Autodesk Fusion 360 part; units mm, degrees
note: some values were not read from the file. Chosen so that the rebuilt part matches the saved one: which bodies a step acts on.
(part 2 of 2)
sketch "Sketch2 (3)" plane through (0, 2, 0) normal (0, 1, 0) x (-1, 0, 0) in component "RFIDShelf"
  circle A0 centre (-31.35, -184.4) radius 3.25
  line L0 (-4, -4.6) -> (-58.7, -4.6)
  line L1 (-58.7, -4.6) -> (-62.7, -8.6)
  line L2 (-62.7, -8.6) -> (-62.7, -50.6)
  line L3 (-62.7, -50.6) -> (-58.7, -54.6)
  line L4 (-58.7, -54.6) -> (-60.7, -54.6)
  line L5 (-60.7, -54.6) -> (-60.7, -95.2)
  line L6 (-60.7, -95.2) -> (-58.7, -95.2)
  line L7 (-58.7, -95.2) -> (-62.7, -99.2)
  line L8 (-62.7, -99.2) -> (-62.7, -111.2)
  line L9 (-62.7, -111.2) -> (-58.7, -115.2)
  line L10 (-58.7, -115.2) -> (-60.7, -115.2)
  line L11 (-60.7, -115.2) -> (-60.7, -119.8)
  line L12 (-60.7, -119.8) -> (-58.7, -119.8)
  line L13 (-58.7, -119.8) -> (-62.7, -123.8)
  line L14 (-62.7, -123.8) -> (-62.7, -145.8)
  line L15 (-62.7, -145.8) -> (-58.7, -149.8)
  line L16 (-58.7, -149.8) -> (-60.7, -149.8)
  line L17 (-60.7, -149.8) -> (-60.7, -154.4)
  line L18 (-60.7, -154.4) -> (-58.7, -154.4)
  line L19 (-58.7, -154.4) -> (-62.7, -158.4)
  line L20 (-62.7, -158.4) -> (-62.7, -214.4)
  line L21 (-62.7, -214.4) -> (0, -214.4)
  line L22 (0, -214.4) -> (0, -158.4)
  line L23 (0, -158.4) -> (-4, -154.4)
  line L24 (-4, -154.4) -> (-2, -154.4)
  line L25 (-2, -154.4) -> (-2, -149.8)
  line L26 (-2, -149.8) -> (-4, -149.8)
  line L27 (-4, -149.8) -> (0, -145.8)
  line L28 (0, -145.8) -> (0, -123.8)
  line L29 (0, -123.8) -> (-4, -119.8)
  line L30 (-4, -119.8) -> (-2, -119.8)
  line L31 (-2, -119.8) -> (-2, -115.2)
  line L32 (-2, -115.2) -> (-4, -115.2)
  line L33 (-4, -115.2) -> (0, -111.2)
  line L34 (0, -111.2) -> (0, -99.2)
  line L35 (0, -99.2) -> (-4, -95.2)
  line L36 (-4, -95.2) -> (-2, -95.2)
  line L37 (-2, -95.2) -> (-2, -54.6)
  line L38 (-2, -54.6) -> (-4, -54.6)
  line L39 (-4, -54.6) -> (0, -50.6)
  line L40 (0, -50.6) -> (0, -8.6)
  line L41 (0, -8.6) -> (-4, -4.6)
  line L42 (-4, -149.8) -> (-58.7, -149.8) construction
  line L43 (-2.2, -149.8) -> (-60.5, -149.8)
  line L44 (-60.5, -149.8) -> (-60.5, -154)
  line L45 (-60.5, -154) -> (-2.2, -154)
  line L46 (-2.2, -154) -> (-2.2, -149.8)
  line L47 (-31.35, -149.8) -> (-31.35, -154) construction
  line L48 (-2.2, -151.9) -> (-4.2, -151.9) construction
  line L49 (-4.2, -149.8) -> (-4.2, -154)
  line L50 (-31.35, -149.8) -> (-31.35, -154) construction
  line L51 (-60.5, -151.9) -> (-58.5, -151.9) construction
  line L52 (-58.5, -154) -> (-58.5, -149.8)
  line L53 (-4.2, -154) -> (-58.5, -154)
  line L54 (-31.35, -154) -> (-52.59, -154) construction
  line L55 (-31.35, -154) -> (-10.11, -154) construction
  line L56 (-52.59, -154) -> (-52.59, -149.8)
  line L57 (-10.11, -154) -> (-10.11, -149.8)
  dimension "d344" = 58.3
  dimension "d345" = 4.2
  dimension "d346" = 2
  dimension "d347" = 4.2
  dimension "d348" = 2
  dimension "d356" = 21.24
  dimension "d357" = 21.24
  constraint coincident L26.end L27.start
  constraint coincident L15.end L16.start
  constraint horizontal L43
  constraint vertical L44
  constraint horizontal L45
  constraint vertical L46
  constraint coincident L42 L43.start
  constraint midpoint L42 L47.start
  constraint midpoint L45 L47.end
  constraint perpendicular L42 L47
  constraint midpoint L46 L48.start
  constraint perpendicular L46 L48
  constraint coincident L43 L49.start
  constraint coincident L45 L49.end
  constraint perpendicular L43 L49
  constraint coincident L48.end L49
  constraint perpendicular L42 L50
  constraint midpoint L44 L51.start
  constraint perpendicular L44 L51
  constraint coincident L45 L52.start
  constraint coincident L42 L52.end
  constraint perpendicular L42 L52
  constraint coincident L51.end L52
  constraint coincident L49 L53.start
  constraint coincident L52 L53.end
  constraint perpendicular L52 L53
  constraint coincident L47.end L53
  constraint coincident L53 L54.end
  constraint coincident L53 L55.end
  constraint coincident L43 L56.end
  constraint coincident L43 L57.end
  constraint perpendicular L42 L57
  constraint perpendicular L43 L56
  measures "d344" distance of L43.start L43.end
  measures "d345" distance of L43.start L45.end
  measures "d346" distance of L48.start L48.end
  measures "d347" distance of L47.start L47.end
  measures "d348" distance of L51.start L51.end
  measures "d356" distance of L47.end L54.end
  measures "d357" distance of L47.end L55.end
extrude "Extrude2''" add sketch "Sketch2 (3)" along normal blind 82.4 separate body contours L26 L43 L45 L46 L49 | L16 L43 L44 L45 L52 | L43 L45 L53 L56 L57 makes body 14 at (58.5, 56.9333, -152.6) makes body 15 at (2.2, 56.9333, -152.6) makes body 16 at (38.43, 29.4667, -154) in component "RFIDShelf"
extrude "Extrude6" add sketch "Sketch2 (3)" along normal blind 10 contours L43 L45 L49 L53 L57 | L43 L45 L52 L53 L56 bodies 14 15 16 in component "RFIDShelf"
extrude "Extrude7'''" add sketch "Sketch2 (3)" against normal blind 10 from surface at 82.4 contours L43 L45 L49 L53 L57 | L43 L45 L52 L53 L56 bodies 14 in component "RFIDShelf"
sketch "Sketch3 (2)" plane through (0, 84.4, 0) normal (0, 1, 0) x (-1, 0, 0) in component "RFIDShelf"
  line L0 (-2.2, -154) -> (-2.2, -149.8)
  line L1 (-2.2, -149.8) -> (-60.5, -149.8)
  line L2 (-60.5, -149.8) -> (-60.5, -154)
  line L3 (-60.5, -154) -> (-2.2, -154)
  line L4 (1.1849, -152.6692) -> (-2.2, -154)
  line L5 (-8.5, -161.5333) -> (-0.9667, -154)
  line L6 (-8.5, -161.5333) -> (-5.8622, -161.5333) construction
  line L7 (-4.2, -154) -> (-58.5, -154)
  dimension "d358" = 45
  constraint coincident L0.start L3.end
  constraint horizontal L6
  constraint coincident L5.end L7
  measures "d358" angle of L5 L6
sketch "Sketch5 (2)" plane through (0, 0, -149.8) normal (0, 0, 1) x (1, 0, 0) in component "RFIDShelf"
  line L0 (2.2, 2) -> (60.5, 2)
  line L1 (52.59, 12) -> (52.59, 74.4)
  line L2 (60.5, 84.4) -> (2.2, 84.4)
  line L3 (10.11, 74.4) -> (10.11, 12)
  line L4 (46.97, 84.4) -> (46.97, 70.87) construction
  line L5 (46.97, 70.87) -> (58.5, 70.87) construction
  line L6 (58.5, 12) -> (58.5, 74.4) construction
  line L7 (26.75, 84.4) -> (26.75, 28.96) construction
  line L8 (26.75, 28.96) -> (58.5, 28.96) construction
  circle A0 centre (26.75, 28.96) radius 1.7
  circle A1 centre (26.75, 28.96) radius 3
  circle A2 centre (46.97, 70.87) radius 3
  circle A3 centre (46.97, 70.87) radius 1.7
  line L9 (10.11, 12) -> (4.2, 12)
  line L10 (4.2, 12) -> (4.2, 74.4)
  line L11 (4.2, 74.4) -> (10.11, 74.4)
  line L12 (2.2, 84.4) -> (2.2, 2)
  line L13 (60.5, 2) -> (60.5, 84.4)
  line L14 (52.59, 74.4) -> (58.5, 74.4)
  line L15 (58.5, 74.4) -> (58.5, 12)
  line L16 (58.5, 12) -> (52.59, 12)
  dimension "d400" = 13.53
  dimension "d401" = 11.53
  dimension "d402" = 55.44
  dimension "d403" = 31.75
  dimension "d404" = 3.4
  dimension "d405" = 6
  dimension "d406" = 6
  dimension "d407" = 3.4
  constraint coincident L2 L4.start
  constraint perpendicular L2 L4
  constraint perpendicular L4 L5
  constraint coincident L5.end L6
  constraint coincident L2 L7.start
  constraint perpendicular L2 L7
  constraint perpendicular L6 L8
  constraint coincident L6 L8.end
  constraint coincident L7.end L8.start
  constraint coincident L4.end L5.start
  constraint concentric A2 A3
  measures "d400" distance of L4.start L4.end
  measures "d401" distance of L4.end L5.end
  measures "d402" distance of L7.start L7.end
  measures "d403" distance of L7.end L8.end
  measures "d404" diameter of A0
  measures "d405" diameter of A1
  measures "d406" diameter of A2
  measures "d407" diameter of A3
extrude "Extrude4" cut sketch "Sketch5 (2)" against normal up to surface (4.2 mm away) contours A0 | A3 bodies 14 in component "RFIDShelf"
extrude "Extrude5" cut sketch "Sketch5 (2)" against normal blind 3.2 contours A1 | A2 bodies 14 in component "RFIDShelf"
sketch "Sketch7" plane through (0, 2, 0) normal (0, 1, 0) x (-1, 0, 0) in component "Main Case"
  circle A0 centre (-31.35, -184.4) radius 3.25
  line L0 (-4, -4.6) -> (-58.7, -4.6)
  line L1 (-58.7, -4.6) -> (-62.7, -8.6)
  line L2 (-62.7, -8.6) -> (-62.7, -50.6)
  line L3 (-62.7, -50.6) -> (-58.7, -54.6)
  line L4 (-58.7, -54.6) -> (-60.7, -54.6)
  line L5 (-60.7, -54.6) -> (-60.7, -95.2)
  line L6 (-60.7, -95.2) -> (-58.7, -95.2)
  line L7 (-58.7, -95.2) -> (-62.7, -99.2)
  line L8 (-62.7, -99.2) -> (-62.7, -111.2)
  line L9 (-62.7, -111.2) -> (-58.7, -115.2)
  line L10 (-58.7, -115.2) -> (-60.7, -115.2)
  line L11 (-60.7, -115.2) -> (-60.7, -119.8)
  line L12 (-60.7, -119.8) -> (-58.7, -119.8)
  line L13 (-58.7, -119.8) -> (-62.7, -123.8)
  line L14 (-62.7, -123.8) -> (-62.7, -145.8)
  line L15 (-62.7, -145.8) -> (-58.7, -149.8)
  line L16 (-58.7, -149.8) -> (-60.7, -149.8)
  line L17 (-60.7, -149.8) -> (-60.7, -154.4)
  line L18 (-60.7, -154.4) -> (-58.7, -154.4)
  line L19 (-58.7, -154.4) -> (-62.7, -158.4)
  line L20 (-62.7, -158.4) -> (-62.7, -214.4)
  line L21 (-62.7, -214.4) -> (0, -214.4)
  line L22 (0, -214.4) -> (0, -158.4)
  line L23 (0, -158.4) -> (-4, -154.4)
  line L24 (-4, -154.4) -> (-2, -154.4)
  line L25 (-2, -154.4) -> (-2, -149.8)
  line L26 (-2, -149.8) -> (-4, -149.8)
  line L27 (-4, -149.8) -> (0, -145.8)
  line L28 (0, -145.8) -> (0, -123.8)
  line L29 (0, -123.8) -> (-4, -119.8)
  line L30 (-4, -119.8) -> (-2, -119.8)
  line L31 (-2, -119.8) -> (-2, -115.2)
  line L32 (-2, -115.2) -> (-4, -115.2)
  line L33 (-4, -115.2) -> (0, -111.2)
  line L34 (0, -111.2) -> (0, -99.2)
  line L35 (0, -99.2) -> (-4, -95.2)
  line L36 (-4, -95.2) -> (-2, -95.2)
  line L37 (-2, -95.2) -> (-2, -54.6)
  line L38 (-2, -54.6) -> (-4, -54.6)
  line L39 (-4, -54.6) -> (0, -50.6)
  line L40 (0, -50.6) -> (0, -8.6)
  line L41 (0, -8.6) -> (-4, -4.6)
  line L42 (-2, -115.2) -> (0, -115.2) construction
  line L43 (0, -115.2) -> (0, -102.2) construction
  line L44 (0, -102.2) -> (-21.5, -102.2)
  line L45 (-21.5, -102.2) -> (-21.5, -121.2)
  line L46 (-21.5, -121.2) -> (0, -121.2)
  line L47 (-20, -61) -> (-43, -61)
  line L48 (-43, -61) -> (-43, -28)
  line L49 (-43, -28) -> (-20, -28)
  line L50 (-20, -28) -> (-20, -61)
  dimension "d504" = 13
  dimension "d505" = 21.5
  dimension "d506" = 19
  constraint coincident L31.end L32.start
  constraint perpendicular L31 L42
  constraint perpendicular L42 L43
  constraint perpendicular L43 L44
  constraint perpendicular L44 L45
  constraint perpendicular L45 L46
  constraint horizontal L47
  constraint vertical L48
  constraint horizontal L49
  constraint vertical L50
  measures "d504" distance of L42.end L43.end
  measures "d505" distance of L43.end L44.end
  measures "d506" distance of L44.end L45.end
extrude "Extrude13" cut sketch "Sketch4" along normal up to surface (2 mm away) contours L4 L13 L19 L34 L35 L36 L38 L58 L59 L62 L65 L66 bodies 1 in component "Main Case"
extrude "Extrude14" cut sketch "Sketch4" along normal blind 2 contours A7 bodies 1 in component "Main Case"
sketch "Sketch8" plane through (0, 2, 0) normal (0, 1, 0) x (-1, 0, 0) in component "Main Case"
  circle A0 centre (-31.35, -74.9) radius 12.5
  line L0 (-4, -54.6) -> (-58.7, -54.6)
  line L1 (-58.7, -54.6) -> (-60.7, -54.6)
  line L2 (-60.7, -54.6) -> (-60.7, -95.2)
  line L3 (-60.7, -95.2) -> (-58.7, -95.2)
  line L4 (-58.7, -95.2) -> (-62.7, -99.2)
  line L5 (-62.7, -99.2) -> (-62.7, -111.2)
  line L6 (-62.7, -111.2) -> (-58.7, -115.2)
  line L7 (-58.7, -115.2) -> (-60.7, -115.2)
  line L8 (-60.7, -115.2) -> (-60.7, -119.8)
  line L9 (-60.7, -119.8) -> (-58.7, -119.8)
  line L10 (-58.7, -119.8) -> (-62.7, -123.8)
  line L11 (-62.7, -123.8) -> (-62.7, -145.8)
  line L12 (-62.7, -145.8) -> (-58.7, -149.8)
  line L13 (-58.7, -149.8) -> (-60.7, -149.8)
  line L14 (-60.7, -149.8) -> (-60.7, -154.4)
  line L15 (-60.7, -154.4) -> (-58.7, -154.4)
  line L16 (-58.7, -154.4) -> (-62.7, -158.4)
  line L17 (-62.7, -158.4) -> (-62.7, -214.4)
  line L18 (-62.7, -214.4) -> (0, -214.4)
  line L19 (0, -214.4) -> (0, -158.4)
  line L20 (0, -158.4) -> (-4, -154.4)
  line L21 (-4, -154.4) -> (-2, -154.4)
  line L22 (-2, -154.4) -> (-2, -149.8)
  line L23 (-2, -149.8) -> (-4, -149.8)
  line L24 (-4, -149.8) -> (0, -145.8)
  line L25 (0, -145.8) -> (0, -123.8)
  line L26 (0, -123.8) -> (-4, -119.8)
  line L27 (-4, -119.8) -> (-2, -119.8)
  line L28 (-2, -119.8) -> (-2, -115.2)
  line L29 (-2, -115.2) -> (-4, -115.2)
  line L30 (-4, -115.2) -> (0, -111.2)
  line L31 (0, -111.2) -> (0, -99.2)
  line L32 (0, -99.2) -> (-4, -95.2)
  line L33 (-4, -95.2) -> (-2, -95.2)
  line L34 (-2, -95.2) -> (-2, -54.6)
  line L35 (-2, -54.6) -> (-4, -54.6)
  circle A1 centre (-31.35, -184.4) radius 3.25
  line L36 (-4, -119.8) -> (-18.2, -119.8)
  line L37 (-18.2, -119.8) -> (-18.2, -104.8)
  line L38 (-18.2, -104.8) -> (-4, -104.8)
  line L39 (-4, -104.8) -> (-4, -119.8)
  dimension "d516" = 14.2
  dimension "d517" = 15
  constraint coincident L26.end L27.start
  constraint parallel L27 L36
  constraint perpendicular L27 L37
  constraint perpendicular L37 L38
  constraint perpendicular L36 L39
  measures "d516" distance of L26.end L36.end
  measures "d517" distance of L36.end L37.end
extrude "Extrude15" cut sketch "Sketch8" against normal blind 2 contours L36 L37 L38 L39 bodies 1 in component "Main Case"
component "Case Attempt 2" placed x (1, 0, 0) y (0, 1, 0) z (0, 0, 1) at (0, 0, 0)
component "Main Case" placed x (1, 0, 0) y (0, 1, 0) z (0, 0, 1) at (0, 0, 0) in component "Case Attempt 2"
component "Case Lid" placed x (1, 0, 0) y (0, 1, 0) z (0, 0, 1) at (0, 0, 0) in component "Case Attempt 2"
component "UnoShelfV2" placed x (1, 0, 0) y (0, 1, 0) z (0, 0, 1) at (0, 0, 0) in component "Case Attempt 2"
component "BatteryShelf" placed x (1, 0, 0) y (0, 1, 0) z (0, 0, 1) at (0, 0, 0) in component "Case Attempt 2"
component "ConverterShelf" placed x (1, 0, 0) y (0, 1, 0) z (0, 0, 1) at (0, 0, 0) in component "Case Attempt 2"
component "RFIDShelf" placed x (1, 0, 0) y (0, 1, 0) z (0, 0, 1) at (0, 0, 0) in component "Case Attempt 2"
equation "thickness = 2 mm"
equation "width = 54.1 mm"
equation "nanoLength = 78.2 mm"
equation "unoBatteryGap = 50 mm"
equation "unoHeight = 8 mm"
equation "portHeight = 12 mm"
equation "gap = 0.2 mm"
equation "converterRFIDGap = 30 mm"
equation "unoLength = 69 mm"
equation "lowerShelfHeight = 10 mm"
equation "upperShelfHeight = 10 mm"
equation "converterLength = 20 mm"
equation "converterWidth = 20 mm"
equation "converterShelfHeight = 10 mm"
equation "RFIDRoofGap = 60 mm"
equation "batteryLength = 45 mm"
equation "batteryWidth = 26 mm"
equation "batteryHeight = 17 mm"
equation "batteryConverterGap = 20 mm"
equation "d121 = thickness"
equation "d122 = screwHeadWidth + 0.5 * thickness + 2 * gap"
equation "d146 = unoBatteryGap"
equation "d147 = ( 3 * thickness ) + ( 2 * batteryHeight ) + ( gap ) + 2 * gap"
equation "d148 = batteryConverterGap"
equation "d149 = screwHeadWidth + 0.5 * thickness + 2 * gap"
equation "d150 = converterRFIDGap"
equation "d151 = 0.5 * thickness + screwHeadWidth + 2 * gap"
equation "d152 = RFIDRoofGap"
equation "d153 = thickness"
equation "d154 = thickness"
equation "d155 = thickness"
equation "d156 = thickness"
equation "d157 = thickness"
equation "d158 = thickness"
equation "d159 = thickness"
equation "d160 = thickness"
equation "d161 = thickness"
equation "d162 = thickness"
equation "d163 = thickness"
equation "d164 = thickness"
equation "d165 = thickness"
equation "d166 = 4 * thickness + 3 * gap + width"
equation "d167 = -thickness"
equation "d168 = thickness + gap + thickness + nanoLength + thickness"
equation "d170 = thickness"
equation "d172 = thickness + gap + thickness + nanoLength + thickness + gap + thickness"
equation "d175 = thickness"
equation "d176 = thickness"
equation "RFIDPortDiameter = 6.5 mm"
equation "d180 = RFIDPortDiameter"
equation "d183 = 0.5 * unoBatteryGap"
equation "d184 = thickness"
equation "d185 = 0.5 * batteryConverterGap"
equation "d186 = thickness"
equation "d187 = 0.5 * converterRFIDGap"
equation "d188 = thickness"
equation "d189 = 0.5 * RFIDRoofGap"
equation "d190 = thickness"
equation "d191 = thickness * 2"
equation "d195 = thickness"
equation "d197 = -( thickness + gap )"
equation "d198 = thickness"
equation "d219 = 2 * thickness"
equation "d225 = thickness"
equation "unoBottomBoardHeight = 4 mm"
equation "d248 = width + gap + ( 2 * thickness )"
equation "d249 = ( 3 * thickness ) + ( 2 * batteryHeight ) + ( gap )"
equation "d258 = batteryWidth + 0.5 * gap"
equation "d259 = batteryHeight + 0.5 * gap"
equation "d260 = thickness"
equation "d261 = thickness"
equation "d262 = batteryWidth + 0.5 * gap"
equation "d263 = batteryHeight + 0.5 * gap"
equation "d264 = thickness"
equation "d265 = -thickness"
equation "d288 = thickness"
equation "d295 = -batteryLength - thickness"
equation "d297 = batteryWidth / 2"
equation "d298 = thickness"
equation "d300 = thickness * 2"
equation "d303 = -( thickness * 2 )"
equation "converterHeight = 10 mm"
equation "converterPortLength = 14.4 mm"
equation "converterPortHeight = 11 mm"
equation "d309 = width + gap + ( 2 * thickness )"
equation "d310 = screwHeadWidth + 0.5 * thickness"
equation "converterBoardHeight = 3 mm"
equation "converterPortNotchHeight = 1 mm"
equation "converterPortWidth = 9.5 mm"
equation "d344 = 2 * thickness + gap + width"
equation "d345 = 0.5 * thickness + screwHeadWidth"
equation "d346 = thickness"
equation "d347 = 0.5 * thickness + screwHeadWidth"
equation "d348 = thickness"
equation "RFIDBoardHeight = 2 mm"
equation "d356 = 15.24 mm + screwHeadDiameter"
equation "d357 = 15.24 mm + screwHeadDiameter"
equation "screwHeadDiameter = 6 mm"
equation "screwHeadWidth = 3.2 mm"
equation "screwThreadDiameter = 3.4 mm"
equation "d377 = width + thickness * 2 + gap"
equation "d378 = screwHeadWidth + 0.5 * thickness"
equation "d381 = thickness + 0.5 * gap + 66.1 mm"
equation "d382 = thickness + 7.6 mm + 0.5 * gap"
equation "d383 = 35.5 mm + thickness + 0.5 * gap"
equation "d384 = thickness + 0.5 * gap + 66.1 mm"
equation "d385 = screwThreadDiameter"
equation "d386 = screwThreadDiameter"
equation "d387 = screwHeadDiameter"
equation "d388 = screwHeadDiameter"
equation "d392 = screwHeadWidth"
equation "d395 = thickness"
equation "d397 = thickness / 2"
equation "d399 = thickness"
equation "d400 = 11.43 mm + thickness + 0.5 * gap"
equation "d401 = 11.43 mm + 0.5 * gap"
equation "d402 = 53.34 mm + thickness + 0.5 * gap"
equation "d404 = screwThreadDiameter"
equation "d405 = screwHeadDiameter"
equation "d406 = screwHeadDiameter"
equation "d407 = screwThreadDiameter"
equation "d410 = -screwHeadWidth"
equation "d412 = 5 * thickness"
equation "d415 = -5 * thickness"
equation "d417 = thickness + 0.5 * gap"
equation "d418 = thickness + 0.5 * gap"
equation "d420 = converterPortWidth + 2 * thickness + gap"
equation "d423 = 3 * thickness + gap + converterPortLength"
equation "d433 = thickness + gap"
equation "d434 = thickness + gap + 66.16 mm"
equation "d436 = thickness + gap"
equation "d445 = screwThreadDiameter"
equation "d446 = screwHeadDiameter"
equation "d447 = screwThreadDiameter"
equation "d448 = screwHeadDiameter"
equation "d449 = screwThreadDiameter"
equation "d450 = screwHeadDiameter"
equation "d451 = screwThreadDiameter"
equation "d452 = screwHeadDiameter"
equation "d453 = -0.5 * thickness"
equation "d458 = thickness"
equation "d459 = 2 * thickness"
equation "d485 = thickness"
equation "d487 = thickness"
equation "screwThreadLength = 8.4 mm"
equation "d489 = thickness + converterPortHeight + gap"
equation "d490 = thickness * 4"
equation "d491 = 4 * thickness"
equation "d493 = thickness"
equation "d494 = -( gap + converterPortLength + thickness )"
equation "d498 = 0.5 * ( converterPortLength + 0.5 * gap )"
equation "d499 = thickness"
equation "d500 = ( 0.5 * converterPortLength + 0.5 * gap )"
equation "d501 = thickness"
equation "d502 = 2 * thickness"
equation "d504 = thickness + converterPortHeight"
equation "d505 = 2 * thickness + 2 * thickness + converterPortWidth + 2 * thickness"
equation "d506 = thickness + converterPortHeight + 3 * thickness"
equation "d507 = thickness + screwHeadWidth + portHeight"
equation "d511 = thickness"
equation "d516 = 2.5 * gap + 2 * thickness + converterPortWidth + gap"
equation "d517 = 2 * thickness + converterPortHeight"
equation "d520 = thickness + 0.5 * gap + 2.5 mm"
equation "d521 = 14 mm + 0.5 * gap + thickness"
equation "d522 = screwHeadDiameter"
equation "d523 = screwThreadDiameter"
equation "d524 = 14 mm + 1.3 mm + thickness + 0.5 * gap"
equation "d525 = thickness + 0.5 * gap + 2.6 mm"
equation "d526 = screwHeadDiameter"
equation "d527 = screwThreadDiameter"
